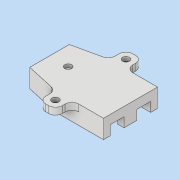
# Autodesk Inventor part: phototransistorMount1
Saved by Autodesk Inventor 2017 (Build 210142000, 142)
## iProperties
Created: 2016-12-12
Part Number: phototransistorMount1
Material: ABS Plastic
Document SubType Name: Modeling
Designer: techn
Density: 1.06 g/cm^3
Appearance: Smooth - White
Author: techn
Autodesk Inventor part; units mm, degrees
ref_plane "YZ Plane" through (0, 0, 0) normal (1, 0, 0) x (0, 1, 0)
ref_plane "XZ Plane" through (0, 0, 0) normal (0, 1, 0) x (-1, 0, 0)
ref_plane "XY Plane" through (0, 0, 0) normal (0, 0, 1) x (1, 0, 0)
sketch "Sketch1" plane through (0, 0, 0) normal (0, 1, 0) x (-1, 0, 0)
  line L0 (0, 0) -> (0, -11.938)
  line L1 (-15.24, 3.3655) -> (-15.24, -15.3035)
  line L2 (0, 0) -> (-15.24, 3.3655)
  line L3 (0, -11.938) -> (-15.24, -15.3035)
  line L4 (-15.24, 3.3655) -> (-19.05, 3.3655)
  line L5 (-19.05, 3.3655) -> (-19.05, 2.0955)
  line L6 (-19.05, 2.0955) -> (-15.24, 2.0955)
  line L7 (-15.24, 2.0955) -> (-15.24, 3.3655)
  line L8 (-15.24, -15.3035) -> (-19.05, -15.3035)
  line L9 (-19.05, -15.3035) -> (-19.05, -14.0335)
  line L10 (-19.05, -14.0335) -> (-15.24, -14.0335)
  line L11 (-15.24, -14.0335) -> (-15.24, -15.3035)
  line L12 (0, 0) -> (0, 3.175)
  line L13 (-15.24, 3.3655) -> (-15.24, 6.5405)
  line L14 (0, -11.938) -> (0, -15.113)
  line L15 (-15.24, -15.3035) -> (-15.24, -18.4785)
  line L16 (-15.24, -18.4785) -> (0, -15.113)
  line L17 (0, 3.175) -> (-15.24, 6.5405)
  line L18 (-15.24, 6.5405) -> (-34.29, 6.5405)
  line L19 (-19.05, 3.3655) -> (-34.29, 3.3655)
  line L20 (-34.29, 3.3655) -> (-34.29, 6.5405)
  line L21 (-15.24, -18.4785) -> (-34.29, -18.4785)
  line L22 (-34.29, -18.4785) -> (-34.29, -15.3035)
  line L23 (-34.29, -15.3035) -> (-19.05, -15.3035)
  line L24 (-34.29, 6.5405) -> (-37.465, 6.5405)
  line L25 (-37.465, 6.5405) -> (-37.465, -18.4785)
  line L26 (-37.465, -18.4785) -> (-34.29, -18.4785)
  line L27 (-34.29, -18.4785) -> (-34.29, 6.5405)
  dimension "d0" = 11.938
  dimension "d1" = 15.24
  dimension "d2" = 18.669
  dimension "d3" = 3.3655
  dimension "d4" = 3.81
  dimension "d5" = 1.27
  dimension "d6" = 3.81
  dimension "d7" = 1.27
  dimension "d8" = 3.175
  dimension "d9" = 3.175
  dimension "d10" = 3.175
  dimension "d11" = 3.175
  dimension "d12" = 19.05
  dimension "d13" = 3.175
  constraints: 56 end point, 7 parallel, 6 perpendicular, 6 vertical, 4 horizontal, 2 point on line
  measures "d0" distance of L0.start L0.end
  measures "d1" distance between parallel lines of L1 L0
  measures "d2" distance of L1.start L1.end
  measures "d3" vertical distance of L1.start L0.start
  measures "d4" distance of L6.end L5.end
  measures "d5" distance of L5.end L4.end
  measures "d6" distance of L9.end L10.end
  measures "d7" distance of L8.end L9.end
  measures "d8" distance of L0.start L12.end
  measures "d9" distance of L1.start L13.end
  measures "d10" distance of L0.end L14.end
  measures "d11" distance of L1.end L15.end
  measures "d12" distance of L13.end L18.end
  measures "d13" distance of L26.end L25.end
extrude "Extrusion1" add sketch "Sketch1" along normal blind 6.985 contours L2 L13 L17 L12 | L14 L16 L15 L3 | L1 L6 L5 L4 | L4 L19 L20 L18 L13 | L8 L9 L10 L1 | L15 L21 L22 L23 L8 | L27 L22 L26 L25 L24 L20
sketch "Sketch2" plane through (0, 6.985, 0) normal (0, 1, 0) x (1, 0, 0)
  line L0 (0, 11.938) -> (15.24, 15.3035) projected
  line L1 (15.24, 15.3035) -> (15.24, 14.0335) projected
  line L2 (15.24, 14.0335) -> (19.05, 14.0335) projected
  line L3 (19.05, 14.0335) -> (19.05, 15.3035) projected
  line L4 (19.05, 15.3035) -> (34.29, 15.3035) projected
  line L5 (34.29, 15.3035) -> (34.29, -3.3655) projected
  line L6 (34.29, -3.3655) -> (19.05, -3.3655) projected
  line L7 (19.05, -3.3655) -> (19.05, -2.0955) projected
  line L8 (19.05, -2.0955) -> (15.24, -2.0955) projected
  line L9 (15.24, -2.0955) -> (15.24, -3.3655) projected
  line L10 (15.24, -3.3655) -> (0, 0) projected
  line L11 (0, 0) -> (0, -3.175) projected
  line L12 (0, -3.175) -> (15.24, -6.5405) projected
  line L13 (15.24, -6.5405) -> (37.465, -6.5405) projected
  line L14 (37.465, -6.5405) -> (37.465, 18.4785) projected
  line L15 (37.465, 18.4785) -> (15.24, 18.4785) projected
  line L16 (15.24, 18.4785) -> (0, 15.113) projected
  line L17 (0, 15.113) -> (0, 11.938) projected
  line L18 (0, 0) -> (0, -3.175) projected
  line L19 (15.24, 18.4785) -> (0, 15.113) projected
  line L20 (0, -3.175) -> (0, 15.113)
  constraints: 2 end point, 1 vertical
extrude "Extrusion2" add sketch "Sketch2" along normal blind 1.5875
sketch "Sketch3" plane through (37.465, 0, 6.5405) normal (1, 0, 0) x (0, 0, -1)
  line L0 (21.844, 0) -> (21.844, 6.985) projected
  line L1 (21.844, 0) -> (3.175, 0) projected
  line L2 (3.175, 0) -> (3.175, 6.985) projected
  line L3 (21.844, 6.985) -> (3.175, 6.985) projected
  line L4 (3.175, 0) -> (3.175, 6.985) projected
  line L5 (3.175, 4.445) -> (9.525, 4.445)
  line L6 (9.525, 4.445) -> (9.525, 0)
  line L7 (9.525, 0) -> (3.175, 0)
  line L8 (3.175, 0) -> (3.175, 4.445)
  line L9 (21.844, 0) -> (21.844, 6.985) projected
  line L10 (21.844, 0) -> (15.494, 0)
  line L11 (15.494, 0) -> (15.494, 4.445)
  line L12 (15.494, 4.445) -> (21.844, 4.445)
  line L13 (21.844, 4.445) -> (21.844, 0)
  line L14 (0, 0) -> (25.019, 0) projected
  point P0 (6.5405, 0)
  dimension "d18" = 6.35
  dimension "d19" = 6.35
  dimension "d20" = 4.445
  dimension "d21" = 4.445
  constraints: 16 end point, 4 parallel, 4 point on line, 2 horizontal, 2 perpendicular
  measures "d18" distance of L6.end L7.end
  measures "d19" distance of L11.end L12.end
  measures "d20" distance of L10.end L11.end
  measures "d21" distance of L5.end L6.end
extrude "Extrusion3" cut sketch "Sketch3" against normal blind 3.175 contours L1 L11 L12 L0 | L1 L2 L5 L6
sketch "Sketch5" plane through (0, 6.985, 0) normal (0, -1, 0) x (1, 0, 0)
  circle A0 centre (8.636, -5.969) radius 1.5875
  line L0 (0, 0) -> (0, 3.175) projected
  line L1 (0, -11.938) -> (0, 0) projected
  dimension "d24" = 3.175
  dimension "d25" = 8.636
  constraints: 1 centre point
  measures "d24" diameter of A0
  measures "d25" distance from line of A0.centre L0
extrude "Extrusion4" cut sketch "Sketch5" against normal blind 25.4
sketch "Sketch6" plane through (0, 8.5725, 0) normal (0, 1, 0) x (1, 0, 0)
  line L0 (37.465, 18.4785) -> (15.24, 18.4785) projected
  line L1 (15.24, -6.5405) -> (37.465, -6.5405) projected
  line L2 (15.24, 18.4785) -> (0, 15.113) projected
  line L3 (15.24, 18.4785) -> (22.86, 18.4785)
  line L4 (22.86, 18.4785) -> (22.86, 26.0985)
  line L5 (22.86, 26.0985) -> (15.24, 26.0985)
  line L6 (15.24, 26.0985) -> (15.24, 18.4785)
  line L7 (15.24, -6.5405) -> (22.86, -6.5405)
  line L8 (22.86, -6.5405) -> (22.86, -14.1605)
  line L9 (22.86, -14.1605) -> (15.24, -14.1605)
  line L10 (15.24, -14.1605) -> (15.24, -6.5405)
  point P0 (0, 0)
  dimension "d28" = 7.62
  dimension "d29" = 7.62
  dimension "d30" = 7.62
  dimension "d31" = 7.62
  constraints: 16 end point, 4 parallel, 2 horizontal, 2 perpendicular
  measures "d28" distance of L5.end L4.end
  measures "d29" distance of L4.end L3.end
  measures "d30" distance of L8.end L9.end
  measures "d31" distance of L7.end L8.end
extrude "Extrusion5" add sketch "Sketch6" against normal blind 3.175
sketch "Sketch7" plane through (0, 5.3975, 0) normal (0, -1, 0) x (1, 0, 0)
  line L0 (22.86, 6.5405) -> (15.24, 6.5405) projected
  line L1 (22.86, 6.5405) -> (22.86, 14.1605) projected
  line L2 (22.86, 14.1605) -> (15.24, 14.1605) projected
  line L3 (15.24, 14.1605) -> (15.24, 6.5405) projected
  line L4 (15.24, -18.4785) -> (22.86, -18.4785) projected
  line L5 (15.24, -18.4785) -> (15.24, -26.0985) projected
  line L6 (15.24, -26.0985) -> (22.86, -26.0985) projected
  line L7 (22.86, -26.0985) -> (22.86, -18.4785) projected
  circle A0 centre (19.05, 10.3505) radius 1.5875
  circle A1 centre (19.05, -22.2885) radius 1.5875
  point P0 (0, 0)
  dimension "d34" = 3.175
  dimension "d35" = 3.175
  constraints: 2 centre point
  measures "d34" diameter of A0
  measures "d35" diameter of A1
extrude "Extrusion6" cut sketch "Sketch7" against normal through all contours A0 | A1
chamfer "Chamfer1" distance 1.27 angle 45 2 edges at (17.4625, 5.3975, 10.3505) (17.4625, 5.3975, -22.2885)
fillet "Fillet1" radius 3.175 8 edges at (15.24, 6.985, -26.0985) (22.86, 6.985, -26.0985) (15.24, 6.985, -18.4785) (22.86, 6.985, -18.4785) (15.24, 6.985, 6.5405) (15.24, 6.985, 14.1605) (22.86, 6.985, 14.1605) (22.86, 6.985, 6.5405)
equation "\"d3\" = -0.5 * d0 + 0.5 * d2"
body "Solid1"
